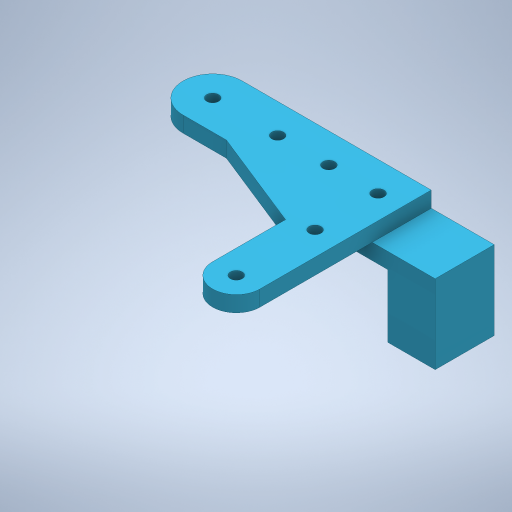
# Autodesk Inventor part: Mounting Bracket 2of4 - Copy2
Saved by Autodesk Inventor 2024 (Build 280153000, 153)
## iProperties
Created: 2019-05-31
Part Number: Mounting Bracket 2of4 - Copy2
Material: Generic
Document SubType Name: Modeling
Designer: cpmcdona
Density: 1 g/cm^3
Appearance: Turquoise
Author: cpmcdona
Autodesk Inventor part; units mm, degrees
ref_plane "YZ Plane" through (0, 0, 0) normal (1, 0, 0) x (0, 1, 0)
ref_plane "XZ Plane" through (0, 0, 0) normal (0, 1, 0) x (-1, 0, 0)
ref_plane "XY Plane" through (0, 0, 0) normal (0, 0, 1) x (1, 0, 0)
sketch "Sketch1" plane through (0, 0, 0) normal (0, 0, 1) x (1, 0, 0)
  circle A0 centre (0, 0) radius 1.5
  circle A1 centre (-42, 0) radius 1.5
  circle A2 centre (0, -36) radius 1.5
  arc A3 (-42, 7.5) -> (-42, -7.5) centre (-42, 0) ccw
  line L0 (-42, 1.5) -> (-42, -1.5)
  arc A4 (-6, -36) -> (6, -36) centre (0, -36) ccw
  line L1 (-42, 7.5) -> (6, 7.5)
  line L2 (6, 7.5) -> (6, -36)
  line L3 (-6, -36) -> (-6, -17.5)
  line L4 (-42, -7.5) -> (-31, -7.5)
  line L5 (-31, -7.5) -> (-6, -17.5)
  dimension "d0" = 3
  dimension "d1" = 3
  dimension "d2" = 3
  dimension "d3" = 15
  dimension "d5" = 15
  dimension "d6" = 12
  dimension "d7" = 48
  constraints: 12 end point, 6 point on circle, 5 centre point, 3 coincident, 2 horizontal, 1 parallel, 1 perpendicular, 1 tangent
  measures "d0" diameter of A0
  measures "d1" diameter of A1
  measures "d2" diameter of A2
  measures "d3" diameter of A3
  measures "d5" distance of L4.start L1.start
  measures "d6" diameter of A4
  measures "d7" distance of L1.start L1.end
extrude "Extrusion1" add sketch "Sketch1" along normal blind 4
sketch "Sketch2" plane through (0, 0, 0) normal (0, 0, -1) x (-1, 0, 0)
  line L0 (6, 7.5) -> (-22, 7.5)
  line L1 (-22, -7.5) -> (6, -7.5)
  line L2 (6, -7.5) -> (6, 7.5)
  line L3 (-22, 7.5) -> (-22, -7.5)
  circle A0 centre (0, 0) radius 1.5
  dimension "d27" = 28
  dimension "d28" = 15
  dimension "d29" = 28
  dimension "d30" = 6
  dimension "d31" = 7.5
  dimension "d32" = 3
  constraints: 8 end point, 1 centre point, 1 coincident, 1 horizontal, 1 parallel, 1 perpendicular
  measures "d27" distance of L0.start L0.end
  measures "d28" distance of L0.end L1.start
  measures "d29" distance of L1.start L1.end
  measures "d30" distance from line of L2 point (0, 0)
  measures "d31" distance from line of L0 point (0, 0)
  measures "d32" diameter of A0
extrude "Extrusion4" add sketch "Sketch2" along normal blind 4
sketch "Sketch5" plane through (0, 0, -4) normal (0, 0, -1) x (-1, 0, 0)
  line L0 (-6, 7.5) -> (-22, 7.5) projected
  line L1 (-22, 7.5) -> (-10, 7.5)
  line L2 (-10, 7.5) -> (-10, -7.5)
  line L3 (-10, -7.5) -> (-22, -7.5)
  line L4 (-22, -7.5) -> (-22, 7.5)
  point P0 (0, 0)
  dimension "d35" = 12
  dimension "d36" = 15
  constraints: 8 end point, 2 equal length, 1 horizontal, 1 parallel
  measures "d35" distance of L2.end L3.end
  measures "d36" distance of L1.end L2.end
extrude "Extrusion5" add sketch "Sketch5" along normal blind 16
shell "Shell2" thickness 4 removed faces 1 at (18, 2.5, -20)
sketch "Sketch6" plane through (0, 0, 0) normal (0, 0, -1) x (-1, 0, 0)
  circle A0 centre (12.5, 0) radius 1.5
  line L0 (6, 7.5) -> (-10, 7.5) projected
  point P0 (0, 0)
  dimension "d40" = 3
  dimension "d41" = 12.5
  dimension "d42" = 7.5
  constraints: 1 centre point
  measures "d40" diameter of A0
  measures "d41" distance of point (0, 0) A0.centre
  measures "d42" distance from line of L0 A0.centre
sketch "Sketch7" plane through (0, 0, 0) normal (0, 0, -1) x (-1, 0, 0)
  point P0 (0, 0)
extrude "Extrusion6" cut sketch "Sketch6" against normal through all
sketch "Sketch8" plane through (0, 0, 0) normal (0, 0, -1) x (-1, 0, 0)
  circle A0 centre (25.5, 0) radius 1.5
  circle A1 centre (12.5, 0) radius 1.5 projected
  line L0 (6, 7.5) -> (-10, 7.5) projected
  point P0 (0, 0)
  dimension "d45" = 3
  dimension "d46" = 13
  dimension "d47" = 7.5
  constraints: 1 centre point
  measures "d45" diameter of A0
  measures "d46" distance of A1.centre A0.centre
  measures "d47" distance from line of L0 A0.centre
extrude "Extrusion7" cut sketch "Sketch8" against normal through all contours A0
sketch "Sketch9" plane through (0, 0, 0) normal (0, 0, -1) x (-1, 0, 0)
  point P0 (0, 0)
sketch "Sketch10" plane through (0, 0, 0) normal (0, 0, -1) x (-1, 0, 0)
  circle A0 centre (0, -16) radius 1.5
  line L0 (6, -36) -> (6, -17.5) projected
  circle A1 centre (0, -36) radius 1.5 projected
  point P0 (0, 0)
  dimension "d50" = 3
  dimension "d51" = 6
  dimension "d52" = 20
  constraints: 1 centre point
  measures "d50" diameter of A0
  measures "d51" distance from line of L0 A0.centre
  measures "d52" distance of A1.centre A0.centre
extrude "Extrusion8" cut sketch "Sketch10" against normal through all contours A0
body "Solid1"
